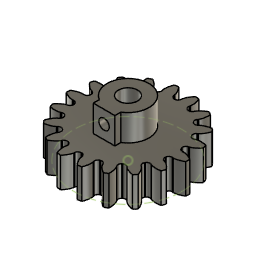
SingleAxisTestJig v42 (Autodesk Fusion 360 archive; units mm, degrees)
design "Drive gear"
description: Spur Gear; Module: 2.000000; Num Teeth: 18; Pressure Angle: 20.000000; Backlash: 0.00 mm
Autodesk Fusion 360 part; units mm, degrees
(part 1 of 2)
sketch "Sketch1" plane through (0, 0, 0) normal (0, 0, 1) x (1, 0, 0) in component "Spur Gear (18 teeth)"
  circle A0 centre (0, 0) radius 15.5492
extrude "Extrude1" add sketch "Sketch1" along normal blind 18 in component "Spur Gear (18 teeth)"
sketch "Sketch2" plane through (0, 0, 0) normal (0, 0, 1) x (1, 0, 0) in component "Spur Gear (18 teeth)"
  spline S0 degree 5 poles (16.8263, -1.7252) (16.8353, -1.7261) (16.8534, -1.7277) (16.8805, -1.7293) (16.9168, -1.7301) (16.9623, -1.7292) (17.0078, -1.7268) (17.0533, -1.7236) (17.0989, -1.7199) (17.1446, -1.7159) (17.1902, -1.7115) (17.2359, -1.7067) (17.2816, -1.7013) (17.3273, -1.6953) (17.373, -1.6885) (17.4187, -1.6812) (17.4644, -1.6733) (17.5101, -1.6649) (17.5558, -1.6561) (17.6016, -1.647) (17.6473, -1.6374) (17.693, -1.6275) (17.7387, -1.6172) (17.7844, -1.6064) (17.8301, -1.5952) (17.8757, -1.5836) (17.9214, -1.5716) (17.967, -1.5592) (18.0127, -1.5465) (18.0583, -1.5335) (18.1039, -1.5201) (18.1494, -1.5063) (18.195, -1.4922) (18.2405, -1.4777) (18.286, -1.463) (18.3315, -1.4478) (18.377, -1.4324) (18.4224, -1.4166) (18.4678, -1.4005) (18.5132, -1.3841) (18.5585, -1.3674) (18.6038, -1.3503) (18.6491, -1.333) (18.6943, -1.3153) (18.7396, -1.2974) (18.7847, -1.2791) (18.8299, -1.2606) (18.875, -1.2418) (18.9201, -1.2226) (18.9651, -1.2032) (19.0101, -1.1835) (19.055, -1.1635) (19.1, -1.1433) (19.1448, -1.1227) (19.1897, -1.1019) (19.2344, -1.0808) (19.2792, -1.0594) (19.3239, -1.0378) (19.3685, -1.0159) (19.4131, -0.9937) (19.4577, -0.9712) (19.5022, -0.9485) (19.5467, -0.9255) (19.5911, -0.9023) (19.6354, -0.8788) (19.6797, -0.855) (19.724, -0.831) (19.7682, -0.8067) (19.8123, -0.7822) (19.8564, -0.7574) (19.9005, -0.7324) (19.9357, -0.7122) (19.962, -0.6969) (19.9796, -0.6867) (19.9884, -0.6815) knots 0 0 0 0 0 0 0.01428571 0.02857143 0.04285714 0.05714286 0.07142857 0.08571429 0.1 0.11428571 0.12857143 0.14285714 0.15714286 0.17142857 0.18571429 0.2 0.21428571 0.22857143 0.24285714 0.25714286 0.27142857 0.28571429 0.3 0.31428571 0.32857143 0.34285714 0.35714286 0.37142857 0.38571429 0.4 0.41428571 0.42857143 0.44285714 0.45714286 0.47142857 0.48571429 0.5 0.51428571 0.52857143 0.54285714 0.55714286 0.57142857 0.58571429 0.6 0.61428571 0.62857143 0.64285714 0.65714286 0.67142857 0.68571429 0.7 0.71428571 0.72857143 0.74285714 0.75714286 0.77142857 0.78571429 0.8 0.81428571 0.82857143 0.84285714 0.85714286 0.87142857 0.88571429 0.9 0.91428571 0.92857143 0.94285714 0.95714286 0.97142857 0.98571429 1 1 1 1 1 1
  spline S1 degree 5 poles (16.8263, 1.7252) (16.8353, 1.7261) (16.8534, 1.7277) (16.8805, 1.7293) (16.9168, 1.7301) (16.9623, 1.7292) (17.0078, 1.7268) (17.0533, 1.7236) (17.0989, 1.7199) (17.1446, 1.7159) (17.1902, 1.7115) (17.2359, 1.7067) (17.2816, 1.7013) (17.3273, 1.6953) (17.373, 1.6885) (17.4187, 1.6812) (17.4644, 1.6733) (17.5101, 1.6649) (17.5558, 1.6561) (17.6016, 1.647) (17.6473, 1.6374) (17.693, 1.6275) (17.7387, 1.6172) (17.7844, 1.6064) (17.8301, 1.5952) (17.8757, 1.5836) (17.9214, 1.5716) (17.967, 1.5592) (18.0127, 1.5465) (18.0583, 1.5335) (18.1039, 1.5201) (18.1494, 1.5063) (18.195, 1.4922) (18.2405, 1.4777) (18.286, 1.463) (18.3315, 1.4478) (18.377, 1.4324) (18.4224, 1.4166) (18.4678, 1.4005) (18.5132, 1.3841) (18.5585, 1.3674) (18.6038, 1.3503) (18.6491, 1.333) (18.6943, 1.3153) (18.7396, 1.2974) (18.7847, 1.2791) (18.8299, 1.2606) (18.875, 1.2418) (18.9201, 1.2226) (18.9651, 1.2032) (19.0101, 1.1835) (19.055, 1.1635) (19.1, 1.1433) (19.1448, 1.1227) (19.1897, 1.1019) (19.2344, 1.0808) (19.2792, 1.0594) (19.3239, 1.0378) (19.3685, 1.0159) (19.4131, 0.9937) (19.4577, 0.9712) (19.5022, 0.9485) (19.5467, 0.9255) (19.5911, 0.9023) (19.6354, 0.8788) (19.6797, 0.855) (19.724, 0.831) (19.7682, 0.8067) (19.8123, 0.7822) (19.8564, 0.7574) (19.9005, 0.7324) (19.9357, 0.7122) (19.962, 0.6969) (19.9796, 0.6867) (19.9884, 0.6815) knots 0 0 0 0 0 0 0.01428571 0.02857143 0.04285714 0.05714286 0.07142857 0.08571429 0.1 0.11428571 0.12857143 0.14285714 0.15714286 0.17142857 0.18571429 0.2 0.21428571 0.22857143 0.24285714 0.25714286 0.27142857 0.28571429 0.3 0.31428571 0.32857143 0.34285714 0.35714286 0.37142857 0.38571429 0.4 0.41428571 0.42857143 0.44285714 0.45714286 0.47142857 0.48571429 0.5 0.51428571 0.52857143 0.54285714 0.55714286 0.57142857 0.58571429 0.6 0.61428571 0.62857143 0.64285714 0.65714286 0.67142857 0.68571429 0.7 0.71428571 0.72857143 0.74285714 0.75714286 0.77142857 0.78571429 0.8 0.81428571 0.82857143 0.84285714 0.85714286 0.87142857 0.88571429 0.9 0.91428571 0.92857143 0.94285714 0.95714286 0.97142857 0.98571429 1 1 1 1 1 1
  arc A0 (19.9884, -0.6815) -> (19.9884, 0.6815) centre (0, 0) ccw
  line L0 (15.4582, -1.5859) -> (16.8263, -1.7252)
  line L1 (15.4582, 1.5859) -> (16.8263, 1.7252)
  line L2 (15.4582, -1.5859) -> (15.4582, 1.5859)
  point P0 (17.0479, -1.7239)
  point P1 (17.2716, -1.7024)
  point P2 (17.4964, -1.6673)
  point P3 (17.7221, -1.6209)
  point P4 (17.9484, -1.5642)
  point P5 (18.1752, -1.4983)
  point P6 (18.4023, -1.4236)
  point P7 (18.6295, -1.3405)
  point P8 (18.8567, -1.2494)
  point P9 (19.0838, -1.1505)
  point P10 (19.3106, -1.0442)
  point P11 (19.5371, -0.9304)
  point P12 (19.763, -0.8095)
  point P13 (17.0479, 1.7239)
  point P14 (17.2716, 1.7024)
  point P15 (17.4964, 1.6673)
  point P16 (17.7221, 1.6209)
  point P17 (17.9484, 1.5642)
  point P18 (18.1752, 1.4983)
  point P19 (18.4023, 1.4236)
  point P20 (18.6295, 1.3405)
  point P21 (18.8567, 1.2494)
  point P22 (19.0838, 1.1505)
  point P23 (19.3106, 1.0442)
  point P24 (19.5371, 0.9304)
  point P25 (19.763, 0.8095)
extrude "Extrude2" add sketch "Sketch2" along normal blind 18 in component "Spur Gear (18 teeth)"
fillet "Fillet1" radius 1.1 2 edges at (15.468, -1.5869, 9) (15.468, 1.5869, 9) in component "Spur Gear (18 teeth)"
pattern_circular "C-Pattern1" count 18 over 360 about axis through (0, 0, 0) along (0, 0, 1) of "Extrude2", "Fillet1" in component "Spur Gear (18 teeth)"
sketch "Sketch3" plane through (0, 0, 0) normal (0, 0, 1) x (1, 0, 0) in component "Spur Gear (18 teeth)"
  circle A0 centre (0, 0) radius 18 construction
extrude "Extrude3" cut 1 faces at (3.3076, 3.9076, 18) along direction (0, 0, -1) blind 8 in component "Spur Gear (18 teeth)"
sketch "Sketch1 (2)" plane through (0, 0, 10) normal (0, 0, 1) x (-1, 0, 0)
  arc A0 (-15.2959, 2.7955) -> (-15.3295, 2.6046) centre (0, 0) ccw
  arc A1 (-16.5253, 1.6945) -> (-15.3295, 2.6046) centre (-16.414, 2.7889) ccw
  line L0 (-16.5253, 1.6945) -> (-16.8263, 1.7252)
  spline S0 degree 3 poles (-19.9884, 0.6815) (-19.5423, 0.9422) (-19.0685, 1.1753) (-17.8142, 1.6475) (-17.3032, 1.701) (-16.9564, 1.7333) (-16.8794, 1.7306) (-16.8263, 1.7252) knots -0.036268 -0.036268 -0.036268 -0.036268 -0.028465 -0.028465 -0.016037 -0.016037 0 0 0 0
  arc A2 (-19.9884, 0.6815) -> (-19.9884, -0.6815) centre (0, 0) ccw
  spline S1 degree 3 poles (-16.8263, -1.7252) (-17.047, -1.7476) (-17.3794, -1.6932) (-17.8324, -1.5988) (-18.0959, -1.5311) (-18.9634, -1.2266) (-19.4935, -0.9707) (-19.9884, -0.6815) knots -0.397989 -0.397989 -0.397989 -0.397989 -0.275735 -0.275735 -0.17197 -0.17197 0 0 0 0
  line L1 (-16.8263, -1.7252) -> (-16.5253, -1.6945)
  arc A3 (-15.3295, -2.6046) -> (-16.5253, -1.6945) centre (-16.414, -2.7889) ccw
  arc A4 (-15.3295, -2.6046) -> (-15.2959, -2.7955) centre (0, 0) ccw
  arc A5 (-16.1083, -4.0597) -> (-15.2959, -2.7955) centre (-16.3779, -2.9932) ccw
  line L2 (-16.1083, -4.0597) -> (-16.4016, -4.1338)
  spline S2 degree 3 poles (-19.016, -6.196) (-18.686, -5.7985) (-18.3205, -5.4174) (-17.3034, -4.5447) (-16.8415, -4.3196) (-16.5266, -4.1706) (-16.4534, -4.1469) (-16.4016, -4.1338) knots -0.036268 -0.036268 -0.036268 -0.036268 -0.028465 -0.028465 -0.016037 -0.016037 0 0 0 0
  arc A6 (-19.016, -6.196) -> (-18.5498, -7.4769) centre (0, 0) ccw
  spline S3 degree 3 poles (-15.2215, -7.376) (-15.4212, -7.4727) (-15.7522, -7.5352) (-16.2101, -7.6014) (-16.4809, -7.6279) (-17.4003, -7.6385) (-17.9858, -7.5794) (-18.5498, -7.4769) knots -0.397989 -0.397989 -0.397989 -0.397989 -0.275735 -0.275735 -0.17197 -0.17197 0 0 0 0
  line L3 (-15.2215, -7.376) -> (-14.9492, -7.2443)
  arc A7 (-13.5142, -7.6905) -> (-14.9492, -7.2443) centre (-14.4702, -8.2346) ccw
  arc A8 (-13.5142, -7.6905) -> (-13.4173, -7.8584) centre (0, 0) ccw
  arc A9 (-13.7484, -9.3242) -> (-13.4173, -7.8584) centre (-14.3665, -8.4143) ccw
  line L4 (-13.7484, -9.3242) -> (-13.9986, -9.4942)
  spline S4 degree 3 poles (-15.7501, -12.3262) (-15.5759, -11.8398) (-15.3628, -11.3566) (-14.7055, -10.1887) (-14.3485, -9.8192) (-14.1035, -9.5715) (-14.0428, -9.5242) (-13.9986, -9.4942) knots -0.036268 -0.036268 -0.036268 -0.036268 -0.028465 -0.028465 -0.016037 -0.016037 0 0 0 0
  arc A10 (-15.7501, -12.3262) -> (-14.8739, -13.3704) centre (0, 0) ccw
  spline S5 degree 3 poles (-11.7808, -12.1373) (-11.9354, -12.2964) (-12.225, -12.4684) (-12.6327, -12.6872) (-12.8781, -12.8047) (-13.7384, -13.1291) (-14.3089, -13.2738) (-14.8739, -13.3704) knots -0.397989 -0.397989 -0.397989 -0.397989 -0.275735 -0.275735 -0.17197 -0.17197 0 0 0 0
  line L5 (-11.7808, -12.1373) -> (-11.5699, -11.9204)
  arc A11 (-10.0689, -11.8489) -> (-11.5699, -11.9204) centre (-10.7812, -12.6871) ccw
  arc A12 (-10.0689, -11.8489) -> (-9.9204, -11.9734) centre (0, 0) ccw
  arc A13 (-9.7302, -13.4641) -> (-9.9204, -11.9734) centre (-10.6222, -12.8205) ccw
  line L6 (-9.7302, -13.4641) -> (-9.9072, -13.7094)
  spline S6 degree 3 poles (-10.5844, -16.9697) (-10.5871, -16.453) (-10.5521, -15.9261) (-10.3339, -14.6038) (-10.1248, -14.1345) (-9.9793, -13.818) (-9.9384, -13.7527) (-9.9072, -13.7094) knots -0.036268 -0.036268 -0.036268 -0.036268 -0.028465 -0.028465 -0.016037 -0.016037 0 0 0 0
  arc A14 (-10.5844, -16.9697) -> (-9.404, -17.6512) centre (0, 0) ccw
  spline S7 degree 3 poles (-6.9191, -15.4345) (-7.01, -15.637) (-7.2234, -15.8976) (-7.5316, -16.2427) (-7.722, -16.4371) (-8.4194, -17.0361) (-8.906, -17.3672) (-9.404, -17.6512) knots -0.397989 -0.397989 -0.397989 -0.397989 -0.275735 -0.275735 -0.17197 -0.17197 0 0 0 0
  line L7 (-6.9191, -15.4345) -> (-6.7952, -15.1586)
  arc A15 (-5.4091, -14.578) -> (-6.7952, -15.1586) centre (-5.7917, -15.6093) ccw
  arc A16 (-5.4091, -14.578) -> (-5.227, -14.6443) centre (0, 0) ccw
  arc A17 (-4.5384, -15.98) -> (-5.227, -14.6443) centre (-5.5968, -15.6803) ccw
  line L8 (-4.5384, -15.98) -> (-4.6208, -16.2711)
  spline S8 degree 3 poles (-4.1421, -19.5664) (-4.3214, -19.0818) (-4.4687, -18.5747) (-4.7159, -17.2575) (-4.6799, -16.745) (-4.6514, -16.3978) (-4.6354, -16.3225) (-4.6208, -16.2711) knots -0.036268 -0.036268 -0.036268 -0.036268 -0.028465 -0.028465 -0.016037 -0.016037 0 0 0 0
  arc A18 (-4.1421, -19.5664) -> (-2.7998, -19.8031) centre (0, 0) ccw
  spline S9 degree 3 poles (-1.2229, -16.8702) (-1.2391, -17.0915) (-1.3504, -17.4094) (-1.5221, -17.8391) (-1.6345, -18.0869) (-2.085, -18.8883) (-2.429, -19.3659) (-2.7998, -19.8031) knots -0.397989 -0.397989 -0.397989 -0.397989 -0.275735 -0.275735 -0.17197 -0.17197 0 0 0 0
  line L9 (-1.2229, -16.8702) -> (-1.2008, -16.5685)
  arc A19 (-0.0969, -15.5489) -> (-1.2008, -16.5685) centre (-0.1037, -16.6489) ccw
  arc A20 (-0.0969, -15.5489) -> (0.0969, -15.5489) centre (0, 0) ccw
  arc A21 (1.2008, -16.5685) -> (0.0969, -15.5489) centre (0.1037, -16.6489) ccw
  line L10 (1.2008, -16.5685) -> (1.2229, -16.8702)
  spline S10 degree 3 poles (2.7998, -19.8031) (2.4656, -19.409) (2.1537, -18.9829) (1.4709, -17.8297) (1.3295, -17.3357) (1.2375, -16.9998) (1.2268, -16.9235) (1.2229, -16.8702) knots -0.036268 -0.036268 -0.036268 -0.036268 -0.028465 -0.028465 -0.016037 -0.016037 0 0 0 0
  arc A22 (2.7998, -19.8031) -> (4.1421, -19.5664) centre (0, 0) ccw
  spline S11 degree 3 poles (4.6208, -16.2711) (4.6813, -16.4846) (4.6854, -16.8214) (4.6711, -17.2838) (4.6502, -17.5551) (4.501, -18.4623) (4.341, -19.0287) (4.1421, -19.5664) knots -0.397989 -0.397989 -0.397989 -0.397989 -0.275735 -0.275735 -0.17197 -0.17197 0 0 0 0
  line L11 (4.6208, -16.2711) -> (4.5384, -15.98)
  arc A23 (5.227, -14.6443) -> (4.5384, -15.98) centre (5.5968, -15.6803) ccw
  arc A24 (5.227, -14.6443) -> (5.4091, -14.578) centre (0, 0) ccw
  arc A25 (6.7952, -15.1586) -> (5.4091, -14.578) centre (5.7917, -15.6093) ccw
  line L12 (6.7952, -15.1586) -> (6.9191, -15.4345)
  spline S12 degree 3 poles (9.404, -17.6512) (8.9552, -17.3952) (8.5164, -17.1015) (7.4803, -16.2513) (7.1785, -15.8356) (6.9771, -15.5513) (6.941, -15.4833) (6.9191, -15.4345) knots -0.036268 -0.036268 -0.036268 -0.036268 -0.028465 -0.028465 -0.016037 -0.016037 0 0 0 0
  arc A26 (9.404, -17.6512) -> (10.5844, -16.9697) centre (0, 0) ccw
  spline S13 degree 3 poles (9.9072, -13.7094) (10.037, -13.8893) (10.1561, -14.2044) (10.3008, -14.6439) (10.3739, -14.906) (10.544, -15.8095) (10.5874, -16.3965) (10.5844, -16.9697) knots -0.397989 -0.397989 -0.397989 -0.397989 -0.275735 -0.275735 -0.17197 -0.17197 0 0 0 0
  line L13 (9.9072, -13.7094) -> (9.7302, -13.4641)
  arc A27 (9.9204, -11.9734) -> (9.7302, -13.4641) centre (10.6222, -12.8205) ccw
  arc A28 (9.9204, -11.9734) -> (10.0689, -11.8489) centre (0, 0) ccw
  arc A29 (11.5699, -11.9204) -> (10.0689, -11.8489) centre (10.7812, -12.6871) ccw
  line L14 (11.5699, -11.9204) -> (11.7808, -12.1373)
  spline S14 degree 3 poles (14.8739, -13.3704) (14.3646, -13.2833) (13.8518, -13.1574) (12.5875, -12.7129) (12.1616, -12.4254) (11.8752, -12.2271) (11.818, -12.1756) (11.7808, -12.1373) knots -0.036268 -0.036268 -0.036268 -0.036268 -0.028465 -0.028465 -0.016037 -0.016037 0 0 0 0
  arc A30 (14.8739, -13.3704) -> (15.7501, -12.3262) centre (0, 0) ccw
  spline S15 degree 3 poles (13.9986, -9.4942) (14.1821, -9.6189) (14.4018, -9.8742) (14.6881, -10.2377) (14.8464, -10.4589) (15.3153, -11.2498) (15.5568, -11.7865) (15.7501, -12.3262) knots -0.397989 -0.397989 -0.397989 -0.397989 -0.275735 -0.275735 -0.17197 -0.17197 0 0 0 0
  line L15 (13.9986, -9.4942) -> (13.7484, -9.3242)
  arc A31 (13.4173, -7.8584) -> (13.7484, -9.3242) centre (14.3665, -8.4143) ccw
  arc A32 (13.4173, -7.8584) -> (13.5142, -7.6905) centre (0, 0) ccw
  arc A33 (14.9492, -7.2443) -> (13.5142, -7.6905) centre (14.4702, -8.2346) ccw
  line L16 (14.9492, -7.2443) -> (15.2215, -7.376)
  spline S16 degree 3 poles (18.5498, -7.4769) (18.0415, -7.5692) (17.5165, -7.6263) (16.1764, -7.641) (15.6779, -7.5165) (15.3409, -7.4282) (15.2696, -7.3993) (15.2215, -7.376) knots -0.036268 -0.036268 -0.036268 -0.036268 -0.028465 -0.028465 -0.016037 -0.016037 0 0 0 0
  arc A34 (18.5498, -7.4769) -> (19.016, -6.196) centre (0, 0) ccw
  spline S17 degree 3 poles (16.4016, -4.1338) (16.6167, -4.1882) (16.9104, -4.353) (17.3038, -4.5967) (17.5283, -4.7504) (18.2393, -5.3332) (18.6499, -5.755) (19.016, -6.196) knots -0.397989 -0.397989 -0.397989 -0.397989 -0.275735 -0.275735 -0.17197 -0.17197 0 0 0 0
  line L17 (16.4016, -4.1338) -> (16.1083, -4.0597)
  arc A35 (15.2959, -2.7955) -> (16.1083, -4.0597) centre (16.3779, -2.9932) ccw
  arc A36 (15.2959, -2.7955) -> (15.3295, -2.6046) centre (0, 0) ccw
  arc A37 (16.5253, -1.6945) -> (15.3295, -2.6046) centre (16.414, -2.7889) ccw
  line L18 (16.5253, -1.6945) -> (16.8263, -1.7252)
  spline S18 degree 3 poles (19.9884, -0.6815) (19.5423, -0.9422) (19.0685, -1.1753) (17.8142, -1.6475) (17.3032, -1.701) (16.9564, -1.7333) (16.8794, -1.7306) (16.8263, -1.7252) knots -0.036268 -0.036268 -0.036268 -0.036268 -0.028465 -0.028465 -0.016037 -0.016037 0 0 0 0
  arc A38 (19.9884, -0.6815) -> (19.9884, 0.6815) centre (0, 0) ccw
  spline S19 degree 3 poles (16.8263, 1.7252) (17.047, 1.7476) (17.3794, 1.6932) (17.8324, 1.5988) (18.0959, 1.5311) (18.9634, 1.2266) (19.4935, 0.9707) (19.9884, 0.6815) knots -0.397989 -0.397989 -0.397989 -0.397989 -0.275735 -0.275735 -0.17197 -0.17197 0 0 0 0
  line L19 (16.8263, 1.7252) -> (16.5253, 1.6945)
  arc A39 (15.3295, 2.6046) -> (16.5253, 1.6945) centre (16.414, 2.7889) ccw
  arc A40 (15.3295, 2.6046) -> (15.2959, 2.7955) centre (0, 0) ccw
  arc A41 (16.1083, 4.0597) -> (15.2959, 2.7955) centre (16.3779, 2.9932) ccw
  line L20 (16.1083, 4.0597) -> (16.4016, 4.1338)
  spline S20 degree 3 poles (19.016, 6.196) (18.686, 5.7985) (18.3205, 5.4174) (17.3034, 4.5447) (16.8415, 4.3196) (16.5266, 4.1706) (16.4534, 4.1469) (16.4016, 4.1338) knots -0.036268 -0.036268 -0.036268 -0.036268 -0.028465 -0.028465 -0.016037 -0.016037 0 0 0 0
  arc A42 (19.016, 6.196) -> (18.5498, 7.4769) centre (0, 0) ccw
  spline S21 degree 3 poles (15.2215, 7.376) (15.4212, 7.4727) (15.7522, 7.5352) (16.2101, 7.6014) (16.4809, 7.6279) (17.4003, 7.6385) (17.9858, 7.5794) (18.5498, 7.4769) knots -0.397989 -0.397989 -0.397989 -0.397989 -0.275735 -0.275735 -0.17197 -0.17197 0 0 0 0
  line L21 (15.2215, 7.376) -> (14.9492, 7.2443)
  arc A43 (13.5142, 7.6905) -> (14.9492, 7.2443) centre (14.4702, 8.2346) ccw
  arc A44 (13.5142, 7.6905) -> (13.4173, 7.8584) centre (0, 0) ccw
  arc A45 (13.7484, 9.3242) -> (13.4173, 7.8584) centre (14.3665, 8.4143) ccw
  line L22 (13.7484, 9.3242) -> (13.9986, 9.4942)
  spline S22 degree 3 poles (15.7501, 12.3262) (15.5759, 11.8398) (15.3628, 11.3566) (14.7055, 10.1887) (14.3485, 9.8192) (14.1035, 9.5715) (14.0428, 9.5242) (13.9986, 9.4942) knots -0.036268 -0.036268 -0.036268 -0.036268 -0.028465 -0.028465 -0.016037 -0.016037 0 0 0 0
  arc A46 (15.7501, 12.3262) -> (14.8739, 13.3704) centre (0, 0) ccw
  spline S23 degree 3 poles (11.7808, 12.1373) (11.9354, 12.2964) (12.225, 12.4684) (12.6327, 12.6872) (12.8781, 12.8047) (13.7384, 13.1291) (14.3089, 13.2738) (14.8739, 13.3704) knots -0.397989 -0.397989 -0.397989 -0.397989 -0.275735 -0.275735 -0.17197 -0.17197 0 0 0 0
  line L23 (11.7808, 12.1373) -> (11.5699, 11.9204)
  arc A47 (10.0689, 11.8489) -> (11.5699, 11.9204) centre (10.7812, 12.6871) ccw
  arc A48 (10.0689, 11.8489) -> (9.9204, 11.9734) centre (0, 0) ccw
  arc A49 (9.7302, 13.4641) -> (9.9204, 11.9734) centre (10.6222, 12.8205) ccw
  line L24 (9.7302, 13.4641) -> (9.9072, 13.7094)
  spline S24 degree 3 poles (10.5844, 16.9697) (10.5871, 16.453) (10.5521, 15.9261) (10.3339, 14.6038) (10.1248, 14.1345) (9.9793, 13.818) (9.9384, 13.7527) (9.9072, 13.7094) knots -0.036268 -0.036268 -0.036268 -0.036268 -0.028465 -0.028465 -0.016037 -0.016037 0 0 0 0
  arc A50 (10.5844, 16.9697) -> (9.404, 17.6512) centre (0, 0) ccw
  spline S25 degree 3 poles (6.9191, 15.4345) (7.01, 15.637) (7.2234, 15.8976) (7.5316, 16.2427) (7.722, 16.4371) (8.4194, 17.0361) (8.906, 17.3672) (9.404, 17.6512) knots -0.397989 -0.397989 -0.397989 -0.397989 -0.275735 -0.275735 -0.17197 -0.17197 0 0 0 0
  line L25 (6.9191, 15.4345) -> (6.7952, 15.1586)
  arc A51 (5.4091, 14.578) -> (6.7952, 15.1586) centre (5.7917, 15.6093) ccw
  arc A52 (5.4091, 14.578) -> (5.227, 14.6443) centre (0, 0) ccw
  arc A53 (4.5384, 15.98) -> (5.227, 14.6443) centre (5.5968, 15.6803) ccw
  line L26 (4.5384, 15.98) -> (4.6208, 16.2711)
  spline S26 degree 3 poles (4.1421, 19.5664) (4.3214, 19.0818) (4.4687, 18.5747) (4.7159, 17.2575) (4.6799, 16.745) (4.6514, 16.3978) (4.6354, 16.3225) (4.6208, 16.2711) knots -0.036268 -0.036268 -0.036268 -0.036268 -0.028465 -0.028465 -0.016037 -0.016037 0 0 0 0
  arc A54 (4.1421, 19.5664) -> (2.7998, 19.8031) centre (0, 0) ccw
  spline S27 degree 3 poles (1.2229, 16.8702) (1.2391, 17.0915) (1.3504, 17.4094) (1.5221, 17.8391) (1.6345, 18.0869) (2.085, 18.8883) (2.429, 19.3659) (2.7998, 19.8031) knots -0.397989 -0.397989 -0.397989 -0.397989 -0.275735 -0.275735 -0.17197 -0.17197 0 0 0 0
  line L27 (1.2229, 16.8702) -> (1.2008, 16.5685)
  arc A55 (0.0969, 15.5489) -> (1.2008, 16.5685) centre (0.1037, 16.6489) ccw
  arc A56 (0.0969, 15.5489) -> (-0.0969, 15.5489) centre (0, 0) ccw
  arc A57 (-1.2008, 16.5685) -> (-0.0969, 15.5489) centre (-0.1037, 16.6489) ccw
  line L28 (-1.2008, 16.5685) -> (-1.2229, 16.8702)
  spline S28 degree 3 poles (-2.7998, 19.8031) (-2.4656, 19.409) (-2.1537, 18.9829) (-1.4709, 17.8297) (-1.3295, 17.3357) (-1.2375, 16.9998) (-1.2268, 16.9235) (-1.2229, 16.8702) knots -0.036268 -0.036268 -0.036268 -0.036268 -0.028465 -0.028465 -0.016037 -0.016037 0 0 0 0
  arc A58 (-2.7998, 19.8031) -> (-4.1421, 19.5664) centre (0, 0) ccw
  spline S29 degree 3 poles (-4.6208, 16.2711) (-4.6813, 16.4846) (-4.6854, 16.8214) (-4.6711, 17.2838) (-4.6502, 17.5551) (-4.501, 18.4623) (-4.341, 19.0287) (-4.1421, 19.5664) knots -0.397989 -0.397989 -0.397989 -0.397989 -0.275735 -0.275735 -0.17197 -0.17197 0 0 0 0
  line L29 (-4.6208, 16.2711) -> (-4.5384, 15.98)
  arc A59 (-5.227, 14.6443) -> (-4.5384, 15.98) centre (-5.5968, 15.6803) ccw
  arc A60 (-5.227, 14.6443) -> (-5.4091, 14.578) centre (0, 0) ccw
  arc A61 (-6.7952, 15.1586) -> (-5.4091, 14.578) centre (-5.7917, 15.6093) ccw
  line L30 (-6.7952, 15.1586) -> (-6.9191, 15.4345)
  spline S30 degree 3 poles (-9.404, 17.6512) (-8.9552, 17.3952) (-8.5164, 17.1015) (-7.4803, 16.2513) (-7.1785, 15.8356) (-6.9771, 15.5513) (-6.941, 15.4833) (-6.9191, 15.4345) knots -0.036268 -0.036268 -0.036268 -0.036268 -0.028465 -0.028465 -0.016037 -0.016037 0 0 0 0
  arc A62 (-9.404, 17.6512) -> (-10.5844, 16.9697) centre (0, 0) ccw
  spline S31 degree 3 poles (-9.9072, 13.7094) (-10.037, 13.8893) (-10.1561, 14.2044) (-10.3008, 14.6439) (-10.3739, 14.906) (-10.544, 15.8095) (-10.5874, 16.3965) (-10.5844, 16.9697) knots -0.397989 -0.397989 -0.397989 -0.397989 -0.275735 -0.275735 -0.17197 -0.17197 0 0 0 0
  line L31 (-9.9072, 13.7094) -> (-9.7302, 13.4641)
  arc A63 (-9.9204, 11.9734) -> (-9.7302, 13.4641) centre (-10.6222, 12.8205) ccw
  arc A64 (-9.9204, 11.9734) -> (-10.0689, 11.8489) centre (0, 0) ccw
  arc A65 (-11.5699, 11.9204) -> (-10.0689, 11.8489) centre (-10.7812, 12.6871) ccw
  line L32 (-11.5699, 11.9204) -> (-11.7808, 12.1373)
  spline S32 degree 3 poles (-14.8739, 13.3704) (-14.3646, 13.2833) (-13.8518, 13.1574) (-12.5875, 12.7129) (-12.1616, 12.4254) (-11.8752, 12.2271) (-11.818, 12.1756) (-11.7808, 12.1373) knots -0.036268 -0.036268 -0.036268 -0.036268 -0.028465 -0.028465 -0.016037 -0.016037 0 0 0 0
  arc A66 (-14.8739, 13.3704) -> (-15.7501, 12.3262) centre (0, 0) ccw
  spline S33 degree 3 poles (-13.9986, 9.4942) (-14.1821, 9.6189) (-14.4018, 9.8742) (-14.6881, 10.2377) (-14.8464, 10.4589) (-15.3153, 11.2498) (-15.5568, 11.7865) (-15.7501, 12.3262) knots -0.397989 -0.397989 -0.397989 -0.397989 -0.275735 -0.275735 -0.17197 -0.17197 0 0 0 0
  line L33 (-13.9986, 9.4942) -> (-13.7484, 9.3242)
  arc A67 (-13.4173, 7.8584) -> (-13.7484, 9.3242) centre (-14.3665, 8.4143) ccw
  arc A68 (-13.4173, 7.8584) -> (-13.5142, 7.6905) centre (0, 0) ccw
  arc A69 (-14.9492, 7.2443) -> (-13.5142, 7.6905) centre (-14.4702, 8.2346) ccw
  line L34 (-14.9492, 7.2443) -> (-15.2215, 7.376)
  spline S34 degree 3 poles (-18.5498, 7.4769) (-18.0415, 7.5692) (-17.5165, 7.6263) (-16.1764, 7.641) (-15.6779, 7.5165) (-15.3409, 7.4282) (-15.2696, 7.3993) (-15.2215, 7.376) knots -0.036268 -0.036268 -0.036268 -0.036268 -0.028465 -0.028465 -0.016037 -0.016037 0 0 0 0
  arc A70 (-18.5498, 7.4769) -> (-19.016, 6.196) centre (0, 0) ccw
  spline S35 degree 3 poles (-16.4016, 4.1338) (-16.6167, 4.1882) (-16.9104, 4.353) (-17.3038, 4.5967) (-17.5283, 4.7504) (-18.2393, 5.3332) (-18.6499, 5.755) (-19.016, 6.196) knots -0.397989 -0.397989 -0.397989 -0.397989 -0.275735 -0.275735 -0.17197 -0.17197 0 0 0 0
  line L35 (-16.4016, 4.1338) -> (-16.1083, 4.0597)
  arc A71 (-15.2959, 2.7955) -> (-16.1083, 4.0597) centre (-16.3779, 2.9932) ccw
  circle A72 centre (0, 0) radius 3.2
  dimension "d11" = 6.4
  constraint coincident A0.centre A2.centre
  measures "d11" diameter of A72
extrude "Extrude4" cut sketch "Sketch1 (2)" against normal blind 2 contours A72 in component "Spur Gear (18 teeth)"
move_face "OffsetFaces1" offset -0.1 1 faces at (-1.1913, 0.6716, 8) in component "Spur Gear (18 teeth)"
sketch "Sketch2 (2)" plane through (0, 0, 10) normal (0, 0, 1) x (-1, 0, 0)
  circle A0 centre (0, 0) radius 3.2
  arc A1 (-15.2959, 2.7955) -> (-15.3295, 2.6046) centre (0, 0) ccw
  arc A2 (-16.5253, 1.6945) -> (-15.3295, 2.6046) centre (-16.414, 2.7889) ccw
  line L0 (-16.5253, 1.6945) -> (-16.8263, 1.7252)
  spline S0 degree 3 poles (-19.9884, 0.6815) (-19.5423, 0.9422) (-19.0685, 1.1753) (-17.8142, 1.6475) (-17.3032, 1.701) (-16.9564, 1.7333) (-16.8794, 1.7306) (-16.8263, 1.7252) knots -0.036268 -0.036268 -0.036268 -0.036268 -0.028465 -0.028465 -0.016037 -0.016037 0 0 0 0
  arc A3 (-19.9884, 0.6815) -> (-19.9884, -0.6815) centre (0, 0) ccw
  spline S1 degree 3 poles (-16.8263, -1.7252) (-17.047, -1.7476) (-17.3794, -1.6932) (-17.8324, -1.5988) (-18.0959, -1.5311) (-18.9634, -1.2266) (-19.4935, -0.9707) (-19.9884, -0.6815) knots -0.397989 -0.397989 -0.397989 -0.397989 -0.275735 -0.275735 -0.17197 -0.17197 0 0 0 0
  line L1 (-16.8263, -1.7252) -> (-16.5253, -1.6945)
  arc A4 (-15.3295, -2.6046) -> (-16.5253, -1.6945) centre (-16.414, -2.7889) ccw
  arc A5 (-15.3295, -2.6046) -> (-15.2959, -2.7955) centre (0, 0) ccw
  arc A6 (-16.1083, -4.0597) -> (-15.2959, -2.7955) centre (-16.3779, -2.9932) ccw
  line L2 (-16.1083, -4.0597) -> (-16.4016, -4.1338)
  spline S2 degree 3 poles (-19.016, -6.196) (-18.686, -5.7985) (-18.3205, -5.4174) (-17.3034, -4.5447) (-16.8415, -4.3196) (-16.5266, -4.1706) (-16.4534, -4.1469) (-16.4016, -4.1338) knots -0.036268 -0.036268 -0.036268 -0.036268 -0.028465 -0.028465 -0.016037 -0.016037 0 0 0 0
  arc A7 (-19.016, -6.196) -> (-18.5498, -7.4769) centre (0, 0) ccw
  spline S3 degree 3 poles (-15.2215, -7.376) (-15.4212, -7.4727) (-15.7522, -7.5352) (-16.2101, -7.6014) (-16.4809, -7.6279) (-17.4003, -7.6385) (-17.9858, -7.5794) (-18.5498, -7.4769) knots -0.397989 -0.397989 -0.397989 -0.397989 -0.275735 -0.275735 -0.17197 -0.17197 0 0 0 0
  line L3 (-15.2215, -7.376) -> (-14.9492, -7.2443)
  arc A8 (-13.5142, -7.6905) -> (-14.9492, -7.2443) centre (-14.4702, -8.2346) ccw
  arc A9 (-13.5142, -7.6905) -> (-13.4173, -7.8584) centre (0, 0) ccw
  arc A10 (-13.7484, -9.3242) -> (-13.4173, -7.8584) centre (-14.3665, -8.4143) ccw
  line L4 (-13.7484, -9.3242) -> (-13.9986, -9.4942)
  spline S4 degree 3 poles (-15.7501, -12.3262) (-15.5759, -11.8398) (-15.3628, -11.3566) (-14.7055, -10.1887) (-14.3485, -9.8192) (-14.1035, -9.5715) (-14.0428, -9.5242) (-13.9986, -9.4942) knots -0.036268 -0.036268 -0.036268 -0.036268 -0.028465 -0.028465 -0.016037 -0.016037 0 0 0 0
  arc A11 (-15.7501, -12.3262) -> (-14.8739, -13.3704) centre (0, 0) ccw
  spline S5 degree 3 poles (-11.7808, -12.1373) (-11.9354, -12.2964) (-12.225, -12.4684) (-12.6327, -12.6872) (-12.8781, -12.8047) (-13.7384, -13.1291) (-14.3089, -13.2738) (-14.8739, -13.3704) knots -0.397989 -0.397989 -0.397989 -0.397989 -0.275735 -0.275735 -0.17197 -0.17197 0 0 0 0
  line L5 (-11.7808, -12.1373) -> (-11.5699, -11.9204)
  arc A12 (-10.0689, -11.8489) -> (-11.5699, -11.9204) centre (-10.7812, -12.6871) ccw
  arc A13 (-10.0689, -11.8489) -> (-9.9204, -11.9734) centre (0, 0) ccw
  arc A14 (-9.7302, -13.4641) -> (-9.9204, -11.9734) centre (-10.6222, -12.8205) ccw
  line L6 (-9.7302, -13.4641) -> (-9.9072, -13.7094)
  spline S6 degree 3 poles (-10.5844, -16.9697) (-10.5871, -16.453) (-10.5521, -15.9261) (-10.3339, -14.6038) (-10.1248, -14.1345) (-9.9793, -13.818) (-9.9384, -13.7527) (-9.9072, -13.7094) knots -0.036268 -0.036268 -0.036268 -0.036268 -0.028465 -0.028465 -0.016037 -0.016037 0 0 0 0
  arc A15 (-10.5844, -16.9697) -> (-9.404, -17.6512) centre (0, 0) ccw
  spline S7 degree 3 poles (-6.9191, -15.4345) (-7.01, -15.637) (-7.2234, -15.8976) (-7.5316, -16.2427) (-7.722, -16.4371) (-8.4194, -17.0361) (-8.906, -17.3672) (-9.404, -17.6512) knots -0.397989 -0.397989 -0.397989 -0.397989 -0.275735 -0.275735 -0.17197 -0.17197 0 0 0 0
  line L7 (-6.9191, -15.4345) -> (-6.7952, -15.1586)
  arc A16 (-5.4091, -14.578) -> (-6.7952, -15.1586) centre (-5.7917, -15.6093) ccw
  arc A17 (-5.4091, -14.578) -> (-5.227, -14.6443) centre (0, 0) ccw
  arc A18 (-4.5384, -15.98) -> (-5.227, -14.6443) centre (-5.5968, -15.6803) ccw
  line L8 (-4.5384, -15.98) -> (-4.6208, -16.2711)
  spline S8 degree 3 poles (-4.1421, -19.5664) (-4.3214, -19.0818) (-4.4687, -18.5747) (-4.7159, -17.2575) (-4.6799, -16.745) (-4.6514, -16.3978) (-4.6354, -16.3225) (-4.6208, -16.2711) knots -0.036268 -0.036268 -0.036268 -0.036268 -0.028465 -0.028465 -0.016037 -0.016037 0 0 0 0
  arc A19 (-4.1421, -19.5664) -> (-2.7998, -19.8031) centre (0, 0) ccw
  spline S9 degree 3 poles (-1.2229, -16.8702) (-1.2391, -17.0915) (-1.3504, -17.4094) (-1.5221, -17.8391) (-1.6345, -18.0869) (-2.085, -18.8883) (-2.429, -19.3659) (-2.7998, -19.8031) knots -0.397989 -0.397989 -0.397989 -0.397989 -0.275735 -0.275735 -0.17197 -0.17197 0 0 0 0
  line L9 (-1.2229, -16.8702) -> (-1.2008, -16.5685)
  arc A20 (-0.0969, -15.5489) -> (-1.2008, -16.5685) centre (-0.1037, -16.6489) ccw
  arc A21 (-0.0969, -15.5489) -> (0.0969, -15.5489) centre (0, 0) ccw
  arc A22 (1.2008, -16.5685) -> (0.0969, -15.5489) centre (0.1037, -16.6489) ccw
  line L10 (1.2008, -16.5685) -> (1.2229, -16.8702)
  spline S10 degree 3 poles (2.7998, -19.8031) (2.4656, -19.409) (2.1537, -18.9829) (1.4709, -17.8297) (1.3295, -17.3357) (1.2375, -16.9998) (1.2268, -16.9235) (1.2229, -16.8702) knots -0.036268 -0.036268 -0.036268 -0.036268 -0.028465 -0.028465 -0.016037 -0.016037 0 0 0 0
  arc A23 (2.7998, -19.8031) -> (4.1421, -19.5664) centre (0, 0) ccw
  spline S11 degree 3 poles (4.6208, -16.2711) (4.6813, -16.4846) (4.6854, -16.8214) (4.6711, -17.2838) (4.6502, -17.5551) (4.501, -18.4623) (4.341, -19.0287) (4.1421, -19.5664) knots -0.397989 -0.397989 -0.397989 -0.397989 -0.275735 -0.275735 -0.17197 -0.17197 0 0 0 0
  line L11 (4.6208, -16.2711) -> (4.5384, -15.98)
  arc A24 (5.227, -14.6443) -> (4.5384, -15.98) centre (5.5968, -15.6803) ccw
  arc A25 (5.227, -14.6443) -> (5.4091, -14.578) centre (0, 0) ccw
  arc A26 (6.7952, -15.1586) -> (5.4091, -14.578) centre (5.7917, -15.6093) ccw
  line L12 (6.7952, -15.1586) -> (6.9191, -15.4345)
  spline S12 degree 3 poles (9.404, -17.6512) (8.9552, -17.3952) (8.5164, -17.1015) (7.4803, -16.2513) (7.1785, -15.8356) (6.9771, -15.5513) (6.941, -15.4833) (6.9191, -15.4345) knots -0.036268 -0.036268 -0.036268 -0.036268 -0.028465 -0.028465 -0.016037 -0.016037 0 0 0 0
  arc A27 (9.404, -17.6512) -> (10.5844, -16.9697) centre (0, 0) ccw
  spline S13 degree 3 poles (9.9072, -13.7094) (10.037, -13.8893) (10.1561, -14.2044) (10.3008, -14.6439) (10.3739, -14.906) (10.544, -15.8095) (10.5874, -16.3965) (10.5844, -16.9697) knots -0.397989 -0.397989 -0.397989 -0.397989 -0.275735 -0.275735 -0.17197 -0.17197 0 0 0 0
  line L13 (9.9072, -13.7094) -> (9.7302, -13.4641)
  arc A28 (9.9204, -11.9734) -> (9.7302, -13.4641) centre (10.6222, -12.8205) ccw
  arc A29 (9.9204, -11.9734) -> (10.0689, -11.8489) centre (0, 0) ccw
  arc A30 (11.5699, -11.9204) -> (10.0689, -11.8489) centre (10.7812, -12.6871) ccw
  line L14 (11.5699, -11.9204) -> (11.7808, -12.1373)
  spline S14 degree 3 poles (14.8739, -13.3704) (14.3646, -13.2833) (13.8518, -13.1574) (12.5875, -12.7129) (12.1616, -12.4254) (11.8752, -12.2271) (11.818, -12.1756) (11.7808, -12.1373) knots -0.036268 -0.036268 -0.036268 -0.036268 -0.028465 -0.028465 -0.016037 -0.016037 0 0 0 0
  arc A31 (14.8739, -13.3704) -> (15.7501, -12.3262) centre (0, 0) ccw
  spline S15 degree 3 poles (13.9986, -9.4942) (14.1821, -9.6189) (14.4018, -9.8742) (14.6881, -10.2377) (14.8464, -10.4589) (15.3153, -11.2498) (15.5568, -11.7865) (15.7501, -12.3262) knots -0.397989 -0.397989 -0.397989 -0.397989 -0.275735 -0.275735 -0.17197 -0.17197 0 0 0 0
  line L15 (13.9986, -9.4942) -> (13.7484, -9.3242)
  arc A32 (13.4173, -7.8584) -> (13.7484, -9.3242) centre (14.3665, -8.4143) ccw
  arc A33 (13.4173, -7.8584) -> (13.5142, -7.6905) centre (0, 0) ccw
  arc A34 (14.9492, -7.2443) -> (13.5142, -7.6905) centre (14.4702, -8.2346) ccw
  line L16 (14.9492, -7.2443) -> (15.2215, -7.376)
  spline S16 degree 3 poles (18.5498, -7.4769) (18.0415, -7.5692) (17.5165, -7.6263) (16.1764, -7.641) (15.6779, -7.5165) (15.3409, -7.4282) (15.2696, -7.3993) (15.2215, -7.376) knots -0.036268 -0.036268 -0.036268 -0.036268 -0.028465 -0.028465 -0.016037 -0.016037 0 0 0 0
  arc A35 (18.5498, -7.4769) -> (19.016, -6.196) centre (0, 0) ccw
  spline S17 degree 3 poles (16.4016, -4.1338) (16.6167, -4.1882) (16.9104, -4.353) (17.3038, -4.5967) (17.5283, -4.7504) (18.2393, -5.3332) (18.6499, -5.755) (19.016, -6.196) knots -0.397989 -0.397989 -0.397989 -0.397989 -0.275735 -0.275735 -0.17197 -0.17197 0 0 0 0
  line L17 (16.4016, -4.1338) -> (16.1083, -4.0597)
  arc A36 (15.2959, -2.7955) -> (16.1083, -4.0597) centre (16.3779, -2.9932) ccw
  arc A37 (15.2959, -2.7955) -> (15.3295, -2.6046) centre (0, 0) ccw
  arc A38 (16.5253, -1.6945) -> (15.3295, -2.6046) centre (16.414, -2.7889) ccw
  line L18 (16.5253, -1.6945) -> (16.8263, -1.7252)
  spline S18 degree 3 poles (19.9884, -0.6815) (19.5423, -0.9422) (19.0685, -1.1753) (17.8142, -1.6475) (17.3032, -1.701) (16.9564, -1.7333) (16.8794, -1.7306) (16.8263, -1.7252) knots -0.036268 -0.036268 -0.036268 -0.036268 -0.028465 -0.028465 -0.016037 -0.016037 0 0 0 0
  arc A39 (19.9884, -0.6815) -> (19.9884, 0.6815) centre (0, 0) ccw
  spline S19 degree 3 poles (16.8263, 1.7252) (17.047, 1.7476) (17.3794, 1.6932) (17.8324, 1.5988) (18.0959, 1.5311) (18.9634, 1.2266) (19.4935, 0.9707) (19.9884, 0.6815) knots -0.397989 -0.397989 -0.397989 -0.397989 -0.275735 -0.275735 -0.17197 -0.17197 0 0 0 0
  line L19 (16.8263, 1.7252) -> (16.5253, 1.6945)
  arc A40 (15.3295, 2.6046) -> (16.5253, 1.6945) centre (16.414, 2.7889) ccw
  arc A41 (15.3295, 2.6046) -> (15.2959, 2.7955) centre (0, 0) ccw
  arc A42 (16.1083, 4.0597) -> (15.2959, 2.7955) centre (16.3779, 2.9932) ccw
  line L20 (16.1083, 4.0597) -> (16.4016, 4.1338)
  spline S20 degree 3 poles (19.016, 6.196) (18.686, 5.7985) (18.3205, 5.4174) (17.3034, 4.5447) (16.8415, 4.3196) (16.5266, 4.1706) (16.4534, 4.1469) (16.4016, 4.1338) knots -0.036268 -0.036268 -0.036268 -0.036268 -0.028465 -0.028465 -0.016037 -0.016037 0 0 0 0
  arc A43 (19.016, 6.196) -> (18.5498, 7.4769) centre (0, 0) ccw
  spline S21 degree 3 poles (15.2215, 7.376) (15.4212, 7.4727) (15.7522, 7.5352) (16.2101, 7.6014) (16.4809, 7.6279) (17.4003, 7.6385) (17.9858, 7.5794) (18.5498, 7.4769) knots -0.397989 -0.397989 -0.397989 -0.397989 -0.275735 -0.275735 -0.17197 -0.17197 0 0 0 0
  line L21 (15.2215, 7.376) -> (14.9492, 7.2443)
  arc A44 (13.5142, 7.6905) -> (14.9492, 7.2443) centre (14.4702, 8.2346) ccw
  arc A45 (13.5142, 7.6905) -> (13.4173, 7.8584) centre (0, 0) ccw
  arc A46 (13.7484, 9.3242) -> (13.4173, 7.8584) centre (14.3665, 8.4143) ccw
  line L22 (13.7484, 9.3242) -> (13.9986, 9.4942)
  spline S22 degree 3 poles (15.7501, 12.3262) (15.5759, 11.8398) (15.3628, 11.3566) (14.7055, 10.1887) (14.3485, 9.8192) (14.1035, 9.5715) (14.0428, 9.5242) (13.9986, 9.4942) knots -0.036268 -0.036268 -0.036268 -0.036268 -0.028465 -0.028465 -0.016037 -0.016037 0 0 0 0
  arc A47 (15.7501, 12.3262) -> (14.8739, 13.3704) centre (0, 0) ccw
  spline S23 degree 3 poles (11.7808, 12.1373) (11.9354, 12.2964) (12.225, 12.4684) (12.6327, 12.6872) (12.8781, 12.8047) (13.7384, 13.1291) (14.3089, 13.2738) (14.8739, 13.3704) knots -0.397989 -0.397989 -0.397989 -0.397989 -0.275735 -0.275735 -0.17197 -0.17197 0 0 0 0
  line L23 (11.7808, 12.1373) -> (11.5699, 11.9204)
  arc A48 (10.0689, 11.8489) -> (11.5699, 11.9204) centre (10.7812, 12.6871) ccw
  arc A49 (10.0689, 11.8489) -> (9.9204, 11.9734) centre (0, 0) ccw
  arc A50 (9.7302, 13.4641) -> (9.9204, 11.9734) centre (10.6222, 12.8205) ccw
  line L24 (9.7302, 13.4641) -> (9.9072, 13.7094)
  spline S24 degree 3 poles (10.5844, 16.9697) (10.5871, 16.453) (10.5521, 15.9261) (10.3339, 14.6038) (10.1248, 14.1345) (9.9793, 13.818) (9.9384, 13.7527) (9.9072, 13.7094) knots -0.036268 -0.036268 -0.036268 -0.036268 -0.028465 -0.028465 -0.016037 -0.016037 0 0 0 0
  arc A51 (10.5844, 16.9697) -> (9.404, 17.6512) centre (0, 0) ccw
  spline S25 degree 3 poles (6.9191, 15.4345) (7.01, 15.637) (7.2234, 15.8976) (7.5316, 16.2427) (7.722, 16.4371) (8.4194, 17.0361) (8.906, 17.3672) (9.404, 17.6512) knots -0.397989 -0.397989 -0.397989 -0.397989 -0.275735 -0.275735 -0.17197 -0.17197 0 0 0 0
  line L25 (6.9191, 15.4345) -> (6.7952, 15.1586)
  arc A52 (5.4091, 14.578) -> (6.7952, 15.1586) centre (5.7917, 15.6093) ccw
  arc A53 (5.4091, 14.578) -> (5.227, 14.6443) centre (0, 0) ccw
  arc A54 (4.5384, 15.98) -> (5.227, 14.6443) centre (5.5968, 15.6803) ccw
  line L26 (4.5384, 15.98) -> (4.6208, 16.2711)
  spline S26 degree 3 poles (4.1421, 19.5664) (4.3214, 19.0818) (4.4687, 18.5747) (4.7159, 17.2575) (4.6799, 16.745) (4.6514, 16.3978) (4.6354, 16.3225) (4.6208, 16.2711) knots -0.036268 -0.036268 -0.036268 -0.036268 -0.028465 -0.028465 -0.016037 -0.016037 0 0 0 0
  arc A55 (4.1421, 19.5664) -> (2.7998, 19.8031) centre (0, 0) ccw
  spline S27 degree 3 poles (1.2229, 16.8702) (1.2391, 17.0915) (1.3504, 17.4094) (1.5221, 17.8391) (1.6345, 18.0869) (2.085, 18.8883) (2.429, 19.3659) (2.7998, 19.8031) knots -0.397989 -0.397989 -0.397989 -0.397989 -0.275735 -0.275735 -0.17197 -0.17197 0 0 0 0
  line L27 (1.2229, 16.8702) -> (1.2008, 16.5685)
  arc A56 (0.0969, 15.5489) -> (1.2008, 16.5685) centre (0.1037, 16.6489) ccw
  arc A57 (0.0969, 15.5489) -> (-0.0969, 15.5489) centre (0, 0) ccw
  arc A58 (-1.2008, 16.5685) -> (-0.0969, 15.5489) centre (-0.1037, 16.6489) ccw
  line L28 (-1.2008, 16.5685) -> (-1.2229, 16.8702)
  spline S28 degree 3 poles (-2.7998, 19.8031) (-2.4656, 19.409) (-2.1537, 18.9829) (-1.4709, 17.8297) (-1.3295, 17.3357) (-1.2375, 16.9998) (-1.2268, 16.9235) (-1.2229, 16.8702) knots -0.036268 -0.036268 -0.036268 -0.036268 -0.028465 -0.028465 -0.016037 -0.016037 0 0 0 0
  arc A59 (-2.7998, 19.8031) -> (-4.1421, 19.5664) centre (0, 0) ccw
  spline S29 degree 3 poles (-4.6208, 16.2711) (-4.6813, 16.4846) (-4.6854, 16.8214) (-4.6711, 17.2838) (-4.6502, 17.5551) (-4.501, 18.4623) (-4.341, 19.0287) (-4.1421, 19.5664) knots -0.397989 -0.397989 -0.397989 -0.397989 -0.275735 -0.275735 -0.17197 -0.17197 0 0 0 0
  line L29 (-4.6208, 16.2711) -> (-4.5384, 15.98)
  arc A60 (-5.227, 14.6443) -> (-4.5384, 15.98) centre (-5.5968, 15.6803) ccw
  arc A61 (-5.227, 14.6443) -> (-5.4091, 14.578) centre (0, 0) ccw
  arc A62 (-6.7952, 15.1586) -> (-5.4091, 14.578) centre (-5.7917, 15.6093) ccw
  line L30 (-6.7952, 15.1586) -> (-6.9191, 15.4345)
  spline S30 degree 3 poles (-9.404, 17.6512) (-8.9552, 17.3952) (-8.5164, 17.1015) (-7.4803, 16.2513) (-7.1785, 15.8356) (-6.9771, 15.5513) (-6.941, 15.4833) (-6.9191, 15.4345) knots -0.036268 -0.036268 -0.036268 -0.036268 -0.028465 -0.028465 -0.016037 -0.016037 0 0 0 0
  arc A63 (-9.404, 17.6512) -> (-10.5844, 16.9697) centre (0, 0) ccw
  spline S31 degree 3 poles (-9.9072, 13.7094) (-10.037, 13.8893) (-10.1561, 14.2044) (-10.3008, 14.6439) (-10.3739, 14.906) (-10.544, 15.8095) (-10.5874, 16.3965) (-10.5844, 16.9697) knots -0.397989 -0.397989 -0.397989 -0.397989 -0.275735 -0.275735 -0.17197 -0.17197 0 0 0 0
  line L31 (-9.9072, 13.7094) -> (-9.7302, 13.4641)
  arc A64 (-9.9204, 11.9734) -> (-9.7302, 13.4641) centre (-10.6222, 12.8205) ccw
  arc A65 (-9.9204, 11.9734) -> (-10.0689, 11.8489) centre (0, 0) ccw
  arc A66 (-11.5699, 11.9204) -> (-10.0689, 11.8489) centre (-10.7812, 12.6871) ccw
  line L32 (-11.5699, 11.9204) -> (-11.7808, 12.1373)
  spline S32 degree 3 poles (-14.8739, 13.3704) (-14.3646, 13.2833) (-13.8518, 13.1574) (-12.5875, 12.7129) (-12.1616, 12.4254) (-11.8752, 12.2271) (-11.818, 12.1756) (-11.7808, 12.1373) knots -0.036268 -0.036268 -0.036268 -0.036268 -0.028465 -0.028465 -0.016037 -0.016037 0 0 0 0
  arc A67 (-14.8739, 13.3704) -> (-15.7501, 12.3262) centre (0, 0) ccw
  spline S33 degree 3 poles (-13.9986, 9.4942) (-14.1821, 9.6189) (-14.4018, 9.8742) (-14.6881, 10.2377) (-14.8464, 10.4589) (-15.3153, 11.2498) (-15.5568, 11.7865) (-15.7501, 12.3262) knots -0.397989 -0.397989 -0.397989 -0.397989 -0.275735 -0.275735 -0.17197 -0.17197 0 0 0 0
  line L33 (-13.9986, 9.4942) -> (-13.7484, 9.3242)
  arc A68 (-13.4173, 7.8584) -> (-13.7484, 9.3242) centre (-14.3665, 8.4143) ccw
  arc A69 (-13.4173, 7.8584) -> (-13.5142, 7.6905) centre (0, 0) ccw
  arc A70 (-14.9492, 7.2443) -> (-13.5142, 7.6905) centre (-14.4702, 8.2346) ccw
  line L34 (-14.9492, 7.2443) -> (-15.2215, 7.376)
  spline S34 degree 3 poles (-18.5498, 7.4769) (-18.0415, 7.5692) (-17.5165, 7.6263) (-16.1764, 7.641) (-15.6779, 7.5165) (-15.3409, 7.4282) (-15.2696, 7.3993) (-15.2215, 7.376) knots -0.036268 -0.036268 -0.036268 -0.036268 -0.028465 -0.028465 -0.016037 -0.016037 0 0 0 0
  arc A71 (-18.5498, 7.4769) -> (-19.016, 6.196) centre (0, 0) ccw
  spline S35 degree 3 poles (-16.4016, 4.1338) (-16.6167, 4.1882) (-16.9104, 4.353) (-17.3038, 4.5967) (-17.5283, 4.7504) (-18.2393, 5.3332) (-18.6499, 5.755) (-19.016, 6.196) knots -0.397989 -0.397989 -0.397989 -0.397989 -0.275735 -0.275735 -0.17197 -0.17197 0 0 0 0
  line L35 (-16.4016, 4.1338) -> (-16.1083, 4.0597)
  arc A72 (-15.2959, 2.7955) -> (-16.1083, 4.0597) centre (-16.3779, 2.9932) ccw
  circle A73 centre (0, 0) radius 7
  dimension "d15" = 14
  constraint coincident A0.centre A1.centre
  measures "d15" diameter of A73
extrude "Extrude5" add sketch "Sketch2 (2)" along normal blind 9 contours A73 in component "Spur Gear (18 teeth)"
sketch "Sketch3 (2)" plane through (0, 0, 0) normal (0, 1, 0) x (1, 0, 0)
  circle A0 centre (0, -14.5) radius 1.75
  dimension "d18" = 3.5
  measures "d18" diameter of A0
extrude "Extrude6" cut sketch "Sketch3 (2)" against normal blind 7 in component "Spur Gear (18 teeth)"
ref_plane "WorkPlane1" through (0, -6, 0) normal (0, 1, 0) x (0, 0, 1)
sketch "Sketch4" plane through (0, -6, 0) normal (0, 1, 0) x (1, 0, 0)
  line L0 (-7, -19) -> (7, -19)
  line L1 (7, -19) -> (7, -10)
  line L2 (7, -10) -> (-7, -10)
  line L3 (-7, -10) -> (-7, -19)
  dimension "d25" = 9
  dimension "d26" = 14
  constraint horizontal L0
  constraint vertical L1
  constraint horizontal L2
  constraint vertical L3
  measures "d25" distance of L0.end L1.end
  measures "d26" distance of L0.start L0.end
extrude "Extrude7" cut sketch "Sketch4" against normal blind 1 in component "Spur Gear (18 teeth)"
move_face "OffsetFaces2" offset -0.2 1 faces at (-0.0797, -5.0637, 19) in component "Spur Gear (18 teeth)"
extrude "Extrude8" add 1 faces at (-1.1913, 0.6716, 7.9) along direction (0, 0, 1) blind 2 in component "Spur Gear (18 teeth)"
extrude "Extrude9" add 1 faces at (0.0436, -6, 10.9183) along direction (0, -1, 0) blind 2 in component "Spur Gear (18 teeth)"
component "Spur Gear (18 teeth)" placed x (1, 0, 0) y (0, 1, 0) z (0, 0, 1) at (0, 0, 0)

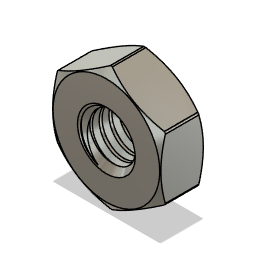
design "M2.5x2mm Hex Nut"
Autodesk Fusion 360 part; units mm, degrees
sketch "Skizze1" plane through (0, 0, 0) normal (0, 0, 1) x (1, 0, 0)
  line L0 (-2.5, -1.4434) -> (0, -2.8868)
  line L1 (0, -2.8868) -> (2.5, -1.4434)
  line L2 (2.5, -1.4434) -> (2.5, 1.4434)
  line L3 (2.5, 1.4434) -> (0, 2.8868)
  line L4 (0, 2.8868) -> (-2.5, 1.4434)
  line L5 (-2.5, 1.4434) -> (-2.5, -1.4434)
  dimension "d3" = 2.5
  constraint vertical L5
  measures "d3" distance of origin L5
extrude "Extrusion1" add sketch "Skizze1" along normal mid plane 2
sketch "Skizze2" plane through (0, 0, 1) normal (0, 0, 1) x (1, 0, 0)
  line L0 (-2.5, 1.4434) -> (-2.5, -1.4434)
  line L1 (-2.5, -1.4434) -> (0, -2.8868)
  line L2 (0, -2.8868) -> (2.5, -1.4434)
  line L3 (2.5, -1.4434) -> (2.5, 1.4434)
  line L4 (2.5, 1.4434) -> (0, 2.8868)
  line L5 (0, 2.8868) -> (-2.5, 1.4434)
hole "Bohrung1" at (0, 0, 1) direction (0, 0, -1) diameter 2.076 end through all
thread "Gewinde1" "ISO Metric profile 2.5 M2.5x0.45 6H" major diameter 2.58 minor diameter 2.0755 pitch 0.45 angle 60 modelled right hand crest width 0.1211 on face at (0.1034, -1.0328, -0.3333) crest through (1.0377, 0, 0.8875)
sketch "Skizze4" plane through (0, 0, 0) normal (1, 0, 0) x (0, 0, -1)
  line L0 (1, 1.4434) -> (1, 2.8868)
  line L1 (1, -2.8868) -> (1, -1.4434)
  line L2 (1, 2.8868) -> (-1, 2.8868)
  line L3 (0.7575, 2.8868) -> (1, 2.4668)
  line L4 (1, 2.8868) -> (0.8181, 2.7818) construction
  line L5 (1, 2.4668) -> (1, 0)
  line L6 (0.7575, 2.8868) -> (0, 2.8868)
  line L7 (0, 1.75) -> (0, 22.5) construction
  line L8 (-0.7575, 2.8868) -> (0, 2.8868)
  line L9 (-0.7575, 2.8868) -> (-1, 2.4668)
  line L10 (-1, 2.4668) -> (-1, 0)
  line L11 (-1, 0) -> (1, 0)
  line L12 (-1, 3.3068) -> (0, 3.3068)
  line L13 (1, 3.3068) -> (0, 3.3068)
  line L14 (1, 3.3068) -> (1.42, 2.5793)
  line L15 (1.42, 2.5793) -> (1.42, -0.42)
  line L16 (-1.42, -0.42) -> (1.42, -0.42)
  line L17 (-1.42, 2.5793) -> (-1.42, -0.42)
  line L18 (-1, 3.3068) -> (-1.42, 2.5793)
  line L19 (-1, 0) -> (-1.42, 0)
  line L20 (1, 0) -> (1.42, 0)
  line L21 (1, -1.4434) -> (1, 1.4434)
  line L22 (-1.75, 0) -> (-22.5, 0)
  dimension "d18" = 0.21
  dimension "d19" = 0.42
  dimension "d23" = 150
  constraint coincident L2 L3.start
  constraint coincident L0 L3.end
  constraint coincident L0.end L2.start
  constraint midpoint L2 L6.end
  constraint symmetric L3.start L7 L8.start
  constraint symmetric L3.end L7 L9.end
  constraint symmetric L5.end L7 L10.end
  constraint symmetric L6.end L7 L8.end
  constraint coincident L17 L19.end
  constraint perpendicular L17 L19
  constraint coincident L15 L20.end
  constraint perpendicular L15 L20
  constraint perpendicular L3 L4
  constraint coincident L3 L4.end
  constraint vertical L10
  constraint collinear L19 L22
  measures "d18" distance of L0.end L4.end
  measures "d23" angle of L3 L5
revolve "Drehen1" cut sketch "Skizze4" angle 360 about axis through (0, 0, 1.75) along (0, 0, 1) contours L0 L2 L5 L6 L8 L9 L10 L12 L13 L14 L15 L17 L18 L19 L20 L21 | L0 L2 L3
fillet "Abrundung1" radius 0.1 6 edges at (2.5, 1.4434, 0) (2.5, -1.4434, 0) (0, -2.8868, 0) (-2.5, -1.4434, 0) (0, 2.8868, 0) (-2.5, 1.4434, 0)
sketch "Skizze5" plane through (0, 0, 0) normal (1, 0, 0) x (0, 0, -1)
  line L0 (-1, 1.3328) -> (-0.7172, 1.05)
  line L1 (-0.7172, 1.05) -> (0, 1.05)
  line L2 (0, 1.75) -> (0, 22.5)
  line L3 (0, 1.05) -> (0, 0) construction
  line L4 (-0.7172, 1.05) -> (-1, 1.05) construction
  line L5 (-1, 1.05) -> (-0.8586, 1.1914) construction
  line L6 (-1, 1.3328) -> (-1, 0)
  line L7 (-1, 0) -> (0, 0)
  line L8 (0.7172, 1.05) -> (0, 1.05)
  line L9 (1, 1.3328) -> (0.7172, 1.05)
  line L10 (1, 1.3328) -> (1, 0)
  line L11 (1, 0) -> (0, 0)
  line L12 (-1, 2.4668) -> (-1, -2.4668)
  dimension "d28" = 1.05
  dimension "d29" = 0.2
  dimension "d31" = 45
  constraint horizontal L1
  constraint coincident L1.end L2
  constraint coincident L3.end L7.end
  constraint coincident L0 L5.end
  constraint perpendicular L0 L5
  constraint symmetric L0.start L2 L9.start
  constraint symmetric L0.end L2 L8.start
  constraint symmetric L1.end L2 L3.start
  constraint symmetric L2 L6.end L10.end
  constraint symmetric L2 L3.end L7.end
  constraint horizontal L7
  constraint vertical L6
  constraint horizontal L4
  constraint coincident L4.end L6
  constraint collinear L6 L12
  measures "d28" distance of L1.end L3.end
  measures "d29" distance of L4.end L5.end
  measures "d31" angle of L0 L6
revolve "Drehen2" cut sketch "Skizze5" angle 360 about axis through (0, 0, 1.75) along (0, 0, 1)
equation "HexWidth = 5 mm" comment "Side-to-side width"
equation "Height = 2 mm"
equation "d3 = HexWidth / 2"
equation "d4 = Height"
equation "ChamferDepth = 0.21 mm" comment "Corner chamfer depth"
equation "ChamferAngle = 30 deg" comment "Corner chamfer angle"
equation "ThreadChamferDepth = 0.2 mm"
equation "d18 = ChamferDepth"
equation "d19 = 2 * ChamferDepth"
equation "SideFillet = 0.1 mm" comment "Fillet of the sides"
equation "d22 = SideFillet"
equation "d23 = 180 deg - ChamferAngle"
equation "ThreadChamferAngle = 45 deg"
equation "CoreDrill = 2.1 mm" comment "Core drill size for the given thread. Used to compute the thread chamfer."
equation "d28 = CoreDrill / 2"
equation "d29 = ThreadChamferDepth"
equation "d31 = ThreadChamferAngle"
named bodies: "Nut"

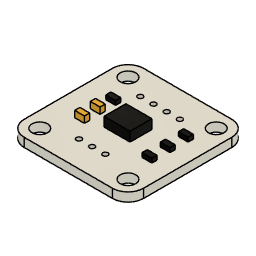
design "AS5600"
Autodesk Fusion 360 part; units mm, degrees